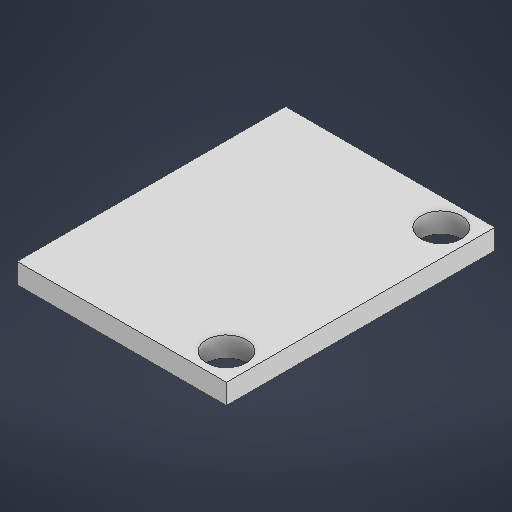
# Autodesk Inventor part: ESP32_C3_SM
Saved by Autodesk Inventor 2026.2 (Build 302298010, 298A)
## iProperties
Created: 2026-05-20
Part Number: ESP32_C3_SM
Material: Generic
Document SubType Name: Modeling
Designer: anton
Density: 1 g/cm^3
Appearance: Default
Author: anton
Autodesk Inventor part; units mm, degrees
ref_plane "YZ Plane" through (0, 0, 0) normal (1, 0, 0) x (0, 1, 0)
ref_plane "XZ Plane" through (0, 0, 0) normal (0, 1, 0) x (-1, 0, 0)
ref_plane "XY Plane" through (0, 0, 0) normal (0, 0, 1) x (1, 0, 0)
sketch "Sketch1" plane through (0, 0, 0) normal (0, 1, 0) x (-1, 0, 0)
  line L0 (0, 0) -> (-15.6, 0)
  line L1 (-15.6, 0) -> (-15.6, -20)
  line L2 (-15.6, -20) -> (0, -20)
  line L3 (0, -20) -> (0, 0)
  line L4 (-15.6, -20) -> (-15.1, -20)
  line L5 (-15.6, -19.5) -> (-15.6, -20)
  circle A0 centre (-13.6, -18) radius 1.5
  circle A1 centre (-13.6, -2) radius 1.5
  dimension "d9" = 15.6
  dimension "d10" = 20
  constraints: 12 end point, 2 centre point, 2 horizontal, 2 parallel, 1 perpendicular
  measures "d9" distance of L2.end L1.end
  measures "d10" distance of L1.end L0.end
extrude "Extrusion3" add sketch "Sketch1" along normal blind 1.5
body "Solid3"
